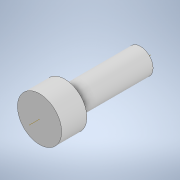
# Autodesk Inventor part: sruba- m4x12
Saved by Autodesk Inventor 2021 (Build 250183000, 183)
## iProperties
Created: 2025-11-29
Part Number: sruba- m4x12
Material: Generic
Document SubType Name: Modeling
Designer: huber
Density: 1 g/cm^3
Appearance: Default
Author: huber
Autodesk Inventor part; units mm, degrees
ref_plane "YZ Plane" through (0, 0, 0) normal (1, 0, 0) x (0, 1, 0)
ref_plane "XZ Plane" through (0, 0, 0) normal (0, 1, 0) x (-1, 0, 0)
ref_plane "XY Plane" through (0, 0, 0) normal (0, 0, 1) x (1, 0, 0)
sketch "Sketch1" plane through (0, 0, 0) normal (1, 0, 0) x (0, 1, 0)
  line L0 (0, 0) -> (3.5, 0)
  line L1 (3.5, 0) -> (3.5, -4)
  line L2 (3.5, -4) -> (2, -4)
  line L3 (2, -4) -> (2, -16)
  line L4 (2, -16) -> (0, -16)
  line L5 (0, -19.2) -> (0, 3.2) projected
  dimension "d1" = 3.5
  dimension "d2" = 16
  dimension "d3" = 2
  dimension "d4" = 4
  constraints: 10 end point, 3 perpendicular, 1 horizontal, 1 parallel, 1 point on line
  measures "d1" distance between parallel lines of L5 L1
  measures "d2" distance between parallel lines of L4 L0
  measures "d3" distance between parallel lines of L5 L3
  measures "d4" distance between parallel lines of L0 L2
revolve "Revolution1" add sketch "Sketch1" angle 360 about axis through (0, 0, -10) along (0, 0, 1)
body "Solid1"
